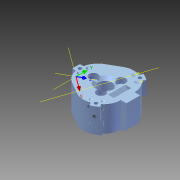
# Autodesk Inventor part: Platform_Base_20mm_Rev2
Saved by Autodesk Inventor 2011 SP2 (Build 150309200, 309)
## iProperties
Created: 2011-03-08
Part Number: Platform_Base_20mm_Rev2
Document SubType Name: Modeling
Designer: sungwook
Density: 2.71 g/cm^3
Material: Aluminum-6061
Mass: 8.63505 g
Surface Area: 22.4979 cm^2
Volume: 3.18636 cm^3
Author: sungwook
Autodesk Inventor part; units mm, degrees
ref_plane "XZ Plane" through (0, 0, 0) normal (0, 1, 0) x (-1, 0, 0)
ref_plane "XY Plane" through (0, 0, 0) normal (0, 0, 1) x (1, 0, 0)
ref_plane "UCS1: YZ Plane" through (-13.0429, 0, 8) normal (0.3420201, 0, -0.9396926) x (0, 1, 0)
sketch "Sketch1" plane through (0, 0, 0) normal (0, 0, 1) x (1, 0, 0)
  circle A0 centre (0, 0) radius 11.5
  dimension "d0" = 23
  constraints: 1 centre point, 1 coincident
  measures "d0" diameter of A0
extrude "Extrusion1" add sketch "Sketch1" along normal blind 12
sketch "Sketch2" plane through (0, 0, 12) normal (0, 0, 1) x (1, 0, 0)
  circle A0 centre (0, 0) radius 11.5 projected
  circle A1 centre (0, 0) radius 10
  line L0 (0, 0) -> (7.6257, 8.6081)
  line L1 (0, 0) -> (3.642, 10.9081)
  line L2 (-18.1349, 0) -> (17.509, 0) projected
  circle A2 centre (3.1669, 9.4853) radius 0.5
  circle A3 centre (6.631, 7.4853) radius 0.5
  line L3 (0, 0) -> (-11.2677, 2.3)
  line L4 (0, 0) -> (-11.2677, -2.3)
  circle A4 centre (-9.798, -2) radius 0.5
  circle A5 centre (-9.798, 2) radius 0.5
  line L5 (0, 0) -> (3.642, -10.9081)
  line L6 (0, 0) -> (7.6257, -8.6081)
  circle A6 centre (6.631, -7.4853) radius 0.5
  circle A7 centre (3.1669, -9.4853) radius 0.5
  dimension "d3" = 20
  dimension "d4" = 48.463
  dimension "d5" = 23.074
  dimension "d6" = 1
  dimension "d7" = 1
  dimension "d178" = 360
  dimension "d425" = 10
  constraints: 12 end point, 7 centre point, 6 point on line, 4 point on circle, 1 coincident, 28 other
  measures "d3" diameter of A1
  measures "d4" angle of L2 L0
  measures "d5" angle of L0 L1
  measures "d6" diameter of A2
  measures "d7" diameter of A3
  measures "d425" distance of A0.centre A3.centre
sketch "Sketch16" plane through (0, 0, 12) normal (0, 0, 1) x (1, 0, 0)
  circle A0 centre (0, 0) radius 11.5 projected
  line L0 (10, 5.6789) -> (10, -5.6789)
  arc A1 (10, -5.6789) -> (10, 5.6789) centre (0, 0) ccw
  dimension "d75" = 10
  constraints: 2 end point, 2 point on circle, 1 centre point, 1 coincident, 1 vertical, 2 other
  measures "d75" distance from line of L0 point (0, 0)
extrude "Extrusion5" cut sketch "Sketch16" against normal through all contours A0 L0 picked at (10.275, -1.294)
pattern_circular "Circular Pattern5" count 3 over 360 about axis through (0, 0, -10) along (0, 0, 1) of "Extrusion5"
fillet "Fillet1" radius 7.62 6 edges at (-9.9181, -5.8208, 6) (-0.0819, -11.4997, 6) (10, -5.6789, 6) (10, 5.6789, 6) (-0.0819, 11.4997, 6) (-9.9181, 5.8208, 6)
sketch "Sketch18" plane through (0, 0, 0) normal (0, 0, -1) x (-1, 0, 0)
  circle A0 centre (0, 0) radius 11.5 projected
  circle A1 centre (0, 0) radius 7
  line L0 (18.1349, 0) -> (-17.509, 0) projected
  point P0 (-7, 0)
  point P1 (-10, -5.6789)
  point P2 (0.0819, -11.4997)
  point P3 (7, 0)
  dimension "d112" = 14
  constraints: 1 coincident, 1 horizontal alignment, 2 other
hole "Attachment Hole M2.5" at (-7, 0, 0) direction (0, 0, 1) diameter 1.7018 depth 4.0132
pattern_circular "Circular Pattern7" count 3 over 360 about axis through (0, 0, -10) along (0, 0, 1) of "Attachment Hole M2.5"
pattern_circular "Circular Pattern8" count 3 over 360 about axis through (0, 0, -10) along (0, 0, 1) of "Attachment Hole M2.5"
ref_plane "Work Plane7" through (6.631, 7.4853, 12) normal (0.7485281, -0.663103, 0) x (-0.663103, -0.7485281, 0)
ref_plane "Work Plane8" through (3.1669, 9.4853, 12) normal (0.9485281, -0.3166929, 0) x (-0.3166929, -0.9485281, 0)
sketch "Sketch21" plane through (6.631, 7.4853, 12) normal (0.7485281, -0.663103, 0) x (-0.663103, -0.7485281, 0)
  line L0 (10, 0) -> (-1.5, 0) projected
  line L1 (0, 0) -> (-1.5543, 7.7083)
  point P0 (10, 12)
  dimension "d147" = 101.4
  constraints: 2 end point, 1 point on line
  measures "d147" angle of L1 L0
hole "Hole12" at (6.631, 7.4853, 12) direction (0.1310672, 0.1479521, -0.9802712) diameter 0.5 end through all countersink diameter 1.5 countersink angle 90
sketch "Sketch22" plane through (6.631, 7.4853, 12) normal (0.7485281, -0.663103, 0) x (-0.663103, -0.7485281, 0)
  line L0 (0, 0) -> (0, 0) projected
  line L1 (0, 0) -> (0, 0) projected
  line L2 (0.1462, 0.5395) -> (-0.3439, 0.4407) projected
  line L3 (0, 0) -> (0.7352, 0.1482) projected
  line L4 (0.7352, 0.1482) -> (0.1462, 0.5395) projected
  line L5 (22.0253, 0) -> (-1.6103, 0) projected
  line L6 (0.7352, 0.1482) -> (2.8954, -1.287)
  line L7 (2.8954, -1.287) -> (0, 0)
  line L8 (2.0956, -10.3929) -> (-3.3737, 16.7318) projected
  point P0 (10, 12)
  constraints: 4 end point, 1 collinear
revolve "Revolution5" cut sketch "Sketch22" angle 360 about axis through (6.631, 7.4853, 12) along (0.1310672, 0.1479521, -0.9802712) contours L6 L5 L3 | L5 L6 L7
sketch "Sketch23" plane through (3.1669, 9.4853, 12) normal (0.9485281, -0.3166929, 0) x (-0.3166929, -0.9485281, 0)
  line L0 (0, 0) -> (-1.0061, 4.9898)
  line L1 (10, 0) -> (-1.5, 0) projected
  point P0 (10, 12)
  dimension "d158" = 101.4
  constraints: 2 end point, 1 point on line
  measures "d158" angle of L0 L1
hole "Hole13" at (3.1669, 9.4853, 12) direction (0.0625967, 0.1874835, -0.9802712) diameter 0.5 end through all countersink diameter 1.5 countersink angle 90
sketch "Sketch24" plane through (3.1669, 9.4853, 12) normal (0.9485281, -0.3166929, 0) x (-0.3166929, -0.9485281, 0)
  line L0 (0.1462, 0.5395) -> (0.7352, 0.1482) projected
  line L1 (0.7352, 0.1482) -> (0, 0) projected
  line L2 (10, 0) -> (-0.58, 0) projected
  line L3 (0.7352, 0.1482) -> (2.2664, -0.8691)
  line L4 (2.2664, -0.8691) -> (0, 0)
  line L5 (-3.2464, 16.1002) -> (1.8788, -9.3177) projected
  point P0 (10, 12)
  constraints: 4 end point, 1 collinear
revolve "Revolution6" cut sketch "Sketch24" angle 360 about axis through (3.4856, 10.4396, 7.0102) along (-0.0625967, -0.1874835, 0.9802712)
pattern_circular "Circular Pattern Top Hole" count 3 over 360 about axis through (0, 0, -10) along (0, 0, 1) of "Hole13", "Revolution6", "Hole12", "Revolution5"
hole "Center Hole" at (0, 0, 12) direction (0, 0, -1) diameter 6 end through all
hole "Center Bottom Bore" at (0, 0, 0) direction (0, 0, 1) diameter 11 depth 2
sketch "Sketch35" plane through (0, 0, 0) normal (0, 0, -1) x (-1, 0, 0)
  line L0 (18.1349, 0) -> (-17.509, 0) projected
  circle A0 centre (-6.1536, 1.5672) radius 1.4986
  circle A1 centre (0, 0) radius 5.5 projected
  circle A2 centre (0, 0) radius 11.5 projected
  line L1 (2.921, 5.0593) -> (0, 0)
  point P0 (-4.3385, 10.6502)
  point P1 (-7.0541, 9.0824)
  dimension "d246" = 2.9972
  dimension "d255" = 6.35
  dimension "d324" = 60
  dimension "d325" = 5.842
  constraints: 2 end point, 1 centre point
  measures "d246" diameter of A0
  measures "d255" distance of A0.centre A1.centre
  measures "d324" angle of L0 L1
  measures "d325" distance of L1.start A1.centre
hole "Jig Hole" at (-2.921, 5.0593, 0) direction (0, 0, 1) diameter 2.9972 depth 5
sketch "Sketch37" plane through (0, 0, 0) normal (0, 0, -1) x (-1, 0, 0)
  circle A0 centre (0, 0) radius 9.64
  line L0 (18.1349, 0) -> (-17.509, 0) projected
  point P0 (9.64, 0)
  dimension "d277" = 19.28
  dimension "d288" = 9.64
  constraints: 1 centre point
  measures "d277" diameter of A0
  measures "d288" distance of A0.centre point (9.64, 0)
hole "PCB Attachment" at (-9.64, 0, 0) direction (0, 0, 1) diameter 1.1938 depth 4.0132
pattern_circular "Circular Pattern11" count 3 over 360 about axis through (0, 0, -10) along (0, 0, 1) of "PCB Attachment"
sketch "Sketch39" plane through (0, 0, 12) normal (0, 0, 1) x (1, 0, 0)
  arc A0 (4.3385, -10.6502) -> (7.0541, -9.0824) centre (0, 0) ccw projected
  circle A1 centre (0, 0) radius 5.2324
  point P0 (-5.2324, 0)
  dimension "d290" = 10.4648
  dimension "d455" = 5.2324
  constraints: 1 coincident, 1 horizontal alignment, 2 other
  measures "d455" distance of A0.centre point (-5.232, 0)
hole "Spring Guide Hole" at (-5.2324, 0, 12) direction (0, 0, -1) diameter 0.4318 end through all counterbore diameter 3.81 counterbore depth 2.54
pattern_circular "Spring r Pattern12" count 3 over 360 about axis through (0, 0, -10) along (0, 0, 1) of "Spring Guide Hole"
sketch "Sketch43" plane through (0, 0, 12) normal (0, 0, 1) x (1, 0, 0)
  line L0 (6.35, 3.81) -> (7.62, 3.81)
  line L1 (7.62, 3.81) -> (7.62, -3.81)
  line L2 (7.62, -3.81) -> (6.35, -3.81)
  line L3 (6.35, -3.81) -> (6.35, 3.81)
  circle A0 centre (0, 0) radius 3 projected
  point P0 (6.35, 0)
  point P1 (-2.6924, -0.0001)
  point P2 (1.3461, 2.3317)
  dimension "d316" = 7.62
  dimension "d317" = 1.27
  dimension "d449" = 6.35
  constraints: 8 end point, 2 parallel, 1 horizontal, 1 midpoint, 1 perpendicular, 1 other
  measures "d316" distance of L1.end L0.end
  measures "d317" distance of L0.end L0.start
  measures "d449" distance from line of L3 point (0, 0)
extrude "PCB Slot" cut sketch "Sketch43" against normal through all contours L0 L1 L2 L3
chamfer "Chamfer3" distance 1.27 angle 45 1 edges at (6.35, 0, 12)
sketch "Sketch48" plane through (0, 0, 0) normal (0, 0, -1) x (-1, 0, 0)
  line L0 (-7.62, 3.81) -> (-6.35, 3.81) projected
  arc A0 (1.4431, 5.3073) -> (3.8747, 3.9034) centre (0, 0) ccw projected
  circle A1 centre (-9.64, 0) radius 0.889
  circle A2 centre (-6.85, 5.5) radius 0.889
  circle A3 centre (-6.85, -5.5) radius 0.889
  line L1 (-7.62, 3.81) -> (-6.35, 3.81)
  line L2 (-6.35, 3.81) -> (-6.35, -3.81)
  line L3 (-6.35, -3.81) -> (-7.62, -3.81)
  line L4 (-7.62, -3.81) -> (-7.62, 3.81)
  line L5 (0, 0) -> (-9.6022, 11.4435)
  line L6 (0, 0) -> (-9.6022, -11.4435)
  arc A4 (-9.6022, 11.4435) -> (-9.6022, -11.4435) centre (0, 0) ccw
  line L7 (18.6392, 0) -> (-20.5347, 0) projected
  circle A5 centre (9.64, 0) radius 0.5969 projected
  line L8 (0, -16.1) -> (0, 16.1) projected
  dimension "d350" = 100
  dimension "d448" = 2.032
  constraints: 12 end point, 4 centre point, 2 point on circle, 1 coincident, 1 point on line, 1 symmetric about line, 1 other
  measures "d350" angle of L6 L5
extrude "Extrusion12" cut sketch "Sketch48" against normal blind 0.635 contours L4 L7 A1 A4 L5 A0 L2 L0 | L4 L3 L2 L7 A0 L6 A4 A1 | L7 A1 | A1 L7 | L7 L6 A0 | A0 L5 L7 | A2 | A3
chamfer "Chamfer4" distance 1.27 angle 45 1 edges at (0, 3, 12)
sketch "Sketch61" plane through (10, -3.0643, 12) normal (1, 0, 0) x (0, 0, -1)
  line L0 (0, 0) -> (11.365, 0)
  line L1 (11.365, 0) -> (11.365, 6.1286)
  line L2 (11.365, 6.1286) -> (0, 6.1286)
  line L3 (0, 6.1286) -> (0, 0)
  point P0 (12, 3.0643)
  constraints: 8 end point, 2 parallel, 1 horizontal, 1 perpendicular
extrude "Extrusion13" add sketch "Sketch61" along normal blind 2.417
hole "Handle LED Mount Holes" at (6.85, 5.5, 0) at (9.64, 0, 0) at (6.85, -5.5, 0) direction (0, 0, 1) diameter 1.1938 depth 3.048
sketch "Sketch63" plane through (0, 0, 0.635) normal (0, 0, -1) x (-1, 0, 0)
  arc A0 (-10.2369, 0) -> (-10.2369, 0) centre (-9.64, 0) ccw projected
  line L0 (-10, 3.0643) -> (-12.417, 3.0643) projected
  line L1 (-12.417, 3.0643) -> (-12.417, -3.0643) projected
  line L2 (-10, -3.0643) -> (-12.417, -3.0643) projected
  arc A1 (-10, -3.0643) -> (-7.3894, -8.8063) centre (-2.38, -3.0643) ccw projected
  line L3 (-7.3894, -8.8063) -> (-3.5353, -4.2132) projected
  arc A2 (-3.5353, 4.2132) -> (-3.5353, -4.2132) centre (0, 0) ccw projected
  line L4 (-3.5353, 4.2132) -> (-7.3894, 8.8063) projected
  arc A3 (-7.3894, 8.8063) -> (-10, 3.0643) centre (-2.38, 3.0643) ccw projected
  circle A4 centre (-6.85, -5.5) radius 0.5969 projected
  circle A5 centre (-6.85, 5.5) radius 0.5969 projected
  line L5 (-7.62, 3.81) -> (-7.62, -3.81) projected
  line L6 (-6.35, 3.81) -> (-7.62, 3.81) projected
  line L7 (-6.35, -3.81) -> (-6.35, 3.81) projected
  line L8 (-7.62, -3.81) -> (-6.35, -3.81) projected
  constraints: 1 coincident
sketch "Sketch64" plane through (0, 0, 12) normal (0, 0, 1) x (1, 0, 0)
  arc A0 (-7.6538, 7.1281) -> (-11.3926, 1.5679) centre (-3.8438, 0.529) ccw projected
  arc A1 (-11.3926, 1.5679) -> (-11.3926, -1.5679) centre (0, 0) ccw projected
  arc A2 (-11.3926, -1.5679) -> (-7.6538, -7.1281) centre (-3.8438, -0.529) ccw projected
  arc A3 (0.7393, 4.2055) -> (-4.0117, 1.4625) centre (0, 0) ccw projected
  line L0 (-25.2834, 0) -> (22.5821, 0) projected
  line L1 (-12.9314, 1.7018) -> (-11.373, 1.7018)
  line L2 (-11.373, -1.7018) -> (-12.9314, -1.7018)
  arc A4 (7.0541, 9.0824) -> (4.3385, 10.6502) centre (0, 0) ccw projected
  arc A5 (4.3385, 10.6502) -> (-2.3462, 10.1924) centre (1.4638, 3.5933) ccw projected
  arc A6 (-4.0117, -1.4625) -> (0.7393, -4.2055) centre (0, 0) ccw projected
  line L3 (0, -22.5821) -> (0, 25.2834) projected
  line L4 (0, 0) -> (7.4747, 16.0297)
  line L5 (7.2545, 10.8393) -> (6.5936, 9.422)
  line L6 (3.6403, 12.5246) -> (2.9597, 11.065)
  line L7 (7.2545, -10.8393) -> (6.5936, -9.422)
  line L8 (3.6403, -12.5246) -> (2.9597, -11.065)
  arc A7 (4.3385, -10.6502) -> (7.0541, -9.0824) centre (0, 0) ccw projected
  arc A8 (-2.3462, -10.1924) -> (4.3385, -10.6502) centre (1.4638, -3.5933) ccw projected
  arc A9 (13.0429, 0) -> (0, -13.0429) centre (0, 0) ccw
  arc A10 (3.6403, -12.5246) -> (7.2545, -10.8393) centre (0, 0) ccw
  dimension "d464" = 3.4036
  dimension "d482" = 25
  dimension "d484" = 3.9878
  dimension "d514" = 13.0429
  constraints: 14 end point, 14 point on circle, 4 symmetric about line, 2 centre point, 2 parallel, 2 point on line, 1 coincident, 1 horizontal, 2 other
  measures "d464" distance between parallel lines of L2 L1
  measures "d482" angle of L4 L3
  measures "d484" distance of L5.start L6.start
  measures "d514" radius of A9
extrude "Extrusion14" add sketch "Sketch64" against normal blind 5.851 contours A0 A1 L0 A9 L1 | A1 A2 L2 A9 L0
pattern_circular "Circular Pattern13" [suppressed]
ref_plane "Work Plane18" through (-13.0429, 0, 12) normal (-1, 0, 0) x (0, -1, 0)
sketch "Sketch65" plane through (-13.0429, 0, 12) normal (-1, 0, 0) x (0, -1, 0)
  line L0 (-1.7018, 0) -> (-1.7018, -5.851) projected
  line L1 (1.7018, 0) -> (1.7018, -5.851) projected
  line L2 (1.7018, 0) -> (-1.7018, 0) projected
  line L3 (1.7018, -5.851) -> (-1.7018, -5.851) projected
  line L4 (0, -14.4003) -> (0, 2.4019) projected
  point P0 (0, -12)
  point P1 (0, -2.5)
  dimension "d470" = 2.5
  constraints: 1 point on line
  measures "d470" distance from line of point (0, -2.5) L2
hole "Hole34" [suppressed]
pattern_circular "Circular Pattern14" [suppressed]
fillet "Fillet3" [suppressed]
ref_plane "Work Plane21" through (-13.0429, 0, 12) normal (-1, 0, 0) x (0, -1, 0)
sketch "Sketch74" plane through (-13.0429, 0, 12) normal (-1, 0, 0) x (0, -1, 0)
  line L0 (1.7018, 0) -> (-1.7018, 0) projected
  line L1 (-1.7018, 0) -> (-1.7018, -5.851) projected
  line L2 (1.7018, 0) -> (1.7018, -5.851) projected
  line L3 (1.7018, -5.851) -> (-1.7018, -5.851) projected
  line L4 (0, -14.4003) -> (0, 2.4019) projected
  point P0 (0, -12)
  point P1 (0, 0)
  point P2 (0, -5.851)
  point P3 (0, -4)
  point P4 (-1.7018, -4)
  dimension "d515" = 4
  constraints: 4 point on line, 2 midpoint, 1 coincident
  measures "d515" distance from line of point (0, -4) L0
sketch "Sketch75" plane through (-13.0429, 0, 8) normal (0.9396926, 0, 0.3420201) x (0.3420201, 0, -0.9396926)
  point P0 (0, 0)
hole "Hole37" at (-13.0429, 0, 8) direction (0.9396926, 0, 0.3420201) diameter 1.1938 depth 4.0132
sketch "Sketch76" plane through (-13.0429, 0, 8) normal (0.9396926, 0, 0.3420201) x (0.3420201, 0, -0.9396926)
  point P0 (0, 0)
hole "Hole38" at (-13.0429, 0, 8) direction (-0.9396926, 0, -0.3420201) diameter 1.1938 end through all
pattern_circular "Circular Pattern16" count 3 over 360 about axis through (0, 0, -10) along (0, 0, 1) of "Hole37", "Hole38", "Extrusion14"
sketch "Sketch77" plane through (0, 0, 0.635) normal (0, 0, -1) x (-1, 0, 0)
  line L0 (-12.417, 3.0643) -> (-11.417, 3.0643)
  line L1 (-11.417, 3.0643) -> (-11.417, -3.0643)
  line L2 (-11.417, -3.0643) -> (-12.417, -3.0643)
  line L3 (-12.417, -3.0643) -> (-12.417, 3.0643)
  point P0 (-10, -3.0643)
  dimension "d539" = 1
  constraints: 8 end point, 2 parallel, 1 horizontal, 1 horizontal alignment, 1 perpendicular
  measures "d539" distance between parallel lines of L3 L1
extrude "Extrusion15" [suppressed]
fillet "Fillet4" [suppressed]
fillet "Fillet5" [suppressed]
sketch "Sketch78" plane through (0, 0, 0) normal (0, 0, -1) x (-1, 0, 0)
  arc A0 (-3.5353, -4.2132) -> (3.8747, 3.9034) centre (0, 0) ccw projected
  circle A1 centre (0, 0) radius 11.5
  circle A2 centre (0, 0) radius 19.2455
  constraints: 2 centre point, 2 coincident
extrude "Extrusion16" cut sketch "Sketch78" against normal up to surface (6.149 mm away)
sketch "Sketch79" plane through (0, 0, 12) normal (0, 0, 1) x (1, 0, 0)
  arc A0 (-12.9314, 1.7018) -> (-12.9314, -1.7018) centre (0, 0) ccw projected
  line L0 (0, -16.8697) -> (0, 16.8697) projected
  line L1 (-18.1363, 0) -> (17.5092, 0) projected
  circle A1 centre (-11.3, 0) radius 1
  dimension "d546" = 2
  dimension "d547" = 11.3
  constraints: 1 centre point, 1 point on line
  measures "d546" diameter of A1
  measures "d547" distance of A0.centre A1.centre
hole "Hole39" at (-11.3, 0, 12) direction (0, 0, -1) diameter 1.5 depth 1.7
pattern_circular "Circular Pattern17" count 3 over 360 about axis through (0, 0, -10) along (0, 0, 1) of "Hole39"
ref_plane "Work Plane25" through (3.6381, 10.8965, 12) normal (0.3166929, 0.9485281, 0) x (-0.9485281, 0.3166929, 0)
ref_plane "Work Plane26" through (7.6176, 8.5989, 12) normal (0.663103, 0.7485281, 0) x (-0.7485281, 0.663103, 0)
ref_plane "Work Plane27" through (7.7018, 8.694, 12) normal (0.663103, 0.7485281, 0) x (-0.7485281, 0.663103, 0)
ref_plane "Work Plane28" through (3.6783, 11.017, 12) normal (0.3166929, 0.9485281, 0) x (-0.9485281, 0.3166929, 0)
sketch "Sketch85" plane through (7.7018, 8.694, 12) normal (0.663103, 0.7485281, 0) x (-0.7485281, 0.663103, 0)
  ellipse E0 centre (2.3709, -3.5674) end of major axis (2.6831, -4.1356) minor radius 0.5969 projected
  line L0 (4.1078, 0) -> (4.1078, -5.851) projected
  line L1 (4.1078, -5.851) -> (0.634, -5.851) projected
  line L2 (0.634, -5.851) -> (0.634, 0) projected
  line L3 (0.634, 0) -> (1.7428, 0) projected
  line L4 (1.7428, 0) -> (1.7428, -1.7) projected
  line L5 (1.7428, -1.7) -> (2.7772, -1.7) projected
  line L6 (2.7772, -1.7) -> (2.7772, 0) projected
  line L7 (2.7772, 0) -> (4.1078, 0) projected
  point P0 (0, -12)
  point P1 (0, 0)
  point P2 (0, -1.905)
  dimension "d593" = 1.905
  constraints: 1 other
  measures "d593" distance of point (0, -1.905) point (0, 0)
sketch "Sketch86" plane through (3.6783, 11.017, 12) normal (0.3166929, 0.9485281, 0) x (-0.9485281, 0.3166929, 0)
  point P0 (0, -12)
  point P1 (0, 0)
  point P2 (0, -1.905)
  dimension "d594" = 1.905
  measures "d594" distance of point (0, -1.905) point (0, 0)
hole "Hole44" at (7.7018, 8.694, 10.095) direction (-0.663103, -0.7485281, 0) diameter 1.1938 depth 1.651
hole "Hole45" at (3.6783, 11.017, 10.095) direction (-0.3166929, -0.9485281, 0) diameter 1.1938 depth 1.651
pattern_circular "Circular Pattern18" count 3 over 360 about axis through (0, 0, -10) along (0, 0, 1) of "Hole44", "Hole45"
mirror "Mirror8" about plane through (0, 0, 0) normal (0, 1, 0) of "Jig Hole"
sketch "Sketch87" plane through (12.417, -3.0643, 12) normal (1, 0, 0) x (0, 0, -1)
  line L0 (5.851, 0) -> (5.851, 6.1286) projected
  line L1 (5.851, 6.1286) -> (11.365, 6.1286) projected
  line L2 (11.365, 0) -> (11.365, 6.1286) projected
  line L3 (11.365, 0) -> (5.851, 0) projected
  point P0 (12, 3.0643)
extrude "Extrusion17" add sketch "Sketch87" against normal up to surface round surface about axis through (0, 0, 0) along (0, 0, 1) radius 11.5 far side no
chamfer "Chamfer5" [suppressed]
sketch "Sketch88" plane through (12.417, -3.0643, 12) normal (1, 0, 0) x (0, 0, -1)
  line L0 (11.365, 6.1286) -> (0, 6.1286) projected
  line L1 (0, 0) -> (0, 6.1286) projected
  line L2 (11.365, 0) -> (0, 0) projected
  line L3 (11.365, 0) -> (11.365, 6.1286) projected
  point P0 (12, 3.0643)
extrude "Extrusion18" add sketch "Sketch88" along normal blind 0.056
chamfer "Chamfer6" distance 1.016 angle 45 1 edges at (12.473, 0, 0.635)
sketch "Sketch89" plane through (0, 0, 0.635) normal (0, 0, -1) x (-1, 0, 0)
  arc A0 (-10, -3.0643) -> (-7.3894, -8.8063) centre (-2.38, -3.0643) ccw projected
  line L0 (-7.3894, -8.8063) -> (-3.5353, -4.2132) projected
  arc A1 (-3.5353, 4.2132) -> (-3.5353, -4.2132) centre (0, 0) ccw projected
  line L1 (-3.5353, 4.2132) -> (-7.3894, 8.8063) projected
  arc A2 (-7.3894, 8.8063) -> (-10, 3.0643) centre (-2.38, 3.0643) ccw projected
  circle A3 centre (-6.85, -5.5) radius 0.5969 projected
  circle A4 centre (-9.64, 0) radius 0.5969 projected
  circle A5 centre (-6.85, 5.5) radius 0.5969 projected
  line L2 (-7.62, 3.81) -> (-7.62, -3.81) projected
  line L3 (-6.35, 3.81) -> (-7.62, 3.81) projected
  line L4 (-6.35, -3.81) -> (-6.35, 3.81) projected
  line L5 (-7.62, -3.81) -> (-6.35, -3.81) projected
  line L6 (-12.473, -10) -> (-12.473, 10)
  line L7 (-7.3894, -8.8063) -> (-12.473, -10)
  line L8 (-7.3894, 8.8063) -> (-12.473, 10)
  point P0 (-12.473, 0)
  point P1 (-12.473, 0)
  dimension "d622" = 20
  constraints: 6 end point, 2 coincident, 1 midpoint
  measures "d622" distance of L6.end L6.start
equation "\"d0\" = baseOD"
equation "\"d3\" = baseD"
equation "\"d4\" = baseTh0"
equation "\"d5\" = baseTh1"
equation "\"baseD\" = 20"
equation "\"springBaseD\" = 8"
equation "\"baseOD\" = 23"
equation "\"CSpringOD\" = 5.537"
equation "\"lFlexure\" = 1.5"
equation "\"springUnderCut\" = 9.2"
equation "\"GuideRod\" = 2"
equation "\"dMotor\" = 1.44"
equation "\"dM2Y\" = 7.00349"
equation "\"GuideTubingOD\" = 4"
equation "\"springInitL\" = 12.7"
equation "\"springL\" = 30.86629"
equation "\"dM1Xt\" = 6.59227"
equation "\"dM2Yt\" = 5.49055"
equation "\"lFlexureOffset\" = 1.95"
equation "\"springDeform\" = 18.16629"
equation "\"dM1Y\" = 2.34012"
equation "\"dM2Xt\" = -3.67462"
equation "\"topH\" = 21.66629"
equation "\"springLO\" = 33.86629"
equation "\"GuideTubingID\" = 2"
equation "\"dM1X\" = 6.73587"
equation "\"lMotor\" = 22.35"
equation "\"CSpringCD\" = 0.254"
equation "\"dM2X\" = -1.34133"
equation "\"dM1Yt\" = -0.43704"
equation "\"CSpringID\" = 5.029"
equation "\"springTopD\" = 8"
equation "\"springLset\" = 3.5"
equation "\"baseInitD\" = 4"
equation "\"topD\" = 14"
equation "\"topInitD\" = 4"
equation "\"dFlexure\" = 0.38"
equation "\"topTh0\" = 16.60155deg"
equation "\"topTh1\" = 86.796901deg"
equation "\"baseTh0\" = 48.463deg"
equation "\"baseTh1\" = 23.0739deg"
equation "\"newBaseOD\" = 26.0858"
equation "\"lOCT\" = 1473.2"
equation "\"lOCTprobe\" = 1905"
equation "\"OCToffset\" = 365.252"
equation "\"lOCTprobeNorm\" = 1838.452"
equation "\"lOCTprobeNom\" = 1838.452"
equation "\"OCTd1\" = 254"
equation "\"OCTd0\" = 508"
body "Solid1"
